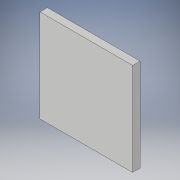
# Autodesk Inventor part: face_part
Saved by Autodesk Inventor 2019 (Build 230136000, 136)
## iProperties
Created: 2019-03-08
Part Number: face_part
Material: Generic
Document SubType Name: Modeling
Designer: Wilson Lab
Density: 1 g/cm^3
Appearance: Default
Author: Wilson Lab
Autodesk Inventor part; units mm, degrees
ref_plane "YZ Plane" through (0, 0, 0) normal (1, 0, 0) x (0, 1, 0)
ref_plane "XZ Plane" through (0, 0, 0) normal (0, 1, 0) x (-1, 0, 0)
ref_plane "XY Plane" through (0, 0, 0) normal (0, 0, 1) x (1, 0, 0)
sketch "Sketch1" plane through (0, 0, 0) normal (0, 0, 1) x (1, 0, 0)
  line L0 (-79, -79) -> (79, -79)
  line L1 (79, -79) -> (79, 79)
  line L2 (79, 79) -> (-79, 79)
  line L3 (-79, 79) -> (-79, -79)
  line L4 (-79, 0) -> (0, 0) construction
  line L5 (0, 0) -> (0, -79) construction
  point P0 (0, -79)
  dimension "d0" = 158
  dimension "d1" = 158
  constraints: 12 end point, 4 midpoint, 2 horizontal, 2 parallel, 2 perpendicular, 2 point on line
  measures "d0" distance of L1.end L2.end
  measures "d1" distance of L0.end L1.end
extrude "Extrusion1" add sketch "Sketch1" along normal blind 12.7
body "Solid1"
